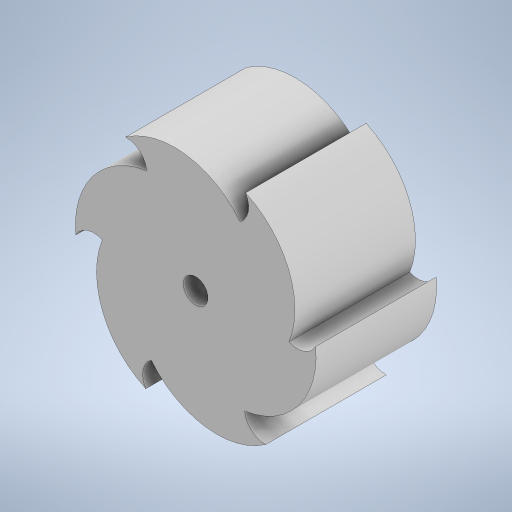
# Autodesk Inventor part: THE_WHEEL
Saved by Autodesk Inventor 2023 (Build 270158000, 158)
## iProperties
Created: 2023-01-26
Part Number: THE_WHEEL
Material: Generic
Document SubType Name: Modeling
Designer: Steven
Density: 1 g/cm^3
Appearance: Default
Author: Steven
Autodesk Inventor part; units mm, degrees
ref_plane "YZ Plane" through (0, 0, 0) normal (1, 0, 0) x (0, 1, 0)
ref_plane "XZ Plane" through (0, 0, 0) normal (0, 1, 0) x (-1, 0, 0)
ref_plane "XY Plane" through (0, 0, 0) normal (0, 0, 1) x (1, 0, 0)
sketch "Sketch1" plane through (0, 0, 0) normal (0, 0, 1) x (1, 0, 0)
  circle A0 centre (0, 0) radius 25.4 construction
  circle A1 centre (0, 0) radius 19.05
  arc A2 (19.0262, -0.952) -> (10.5106, 23.1233) centre (3.175, 6.985) ccw
  arc A3 (8.7227, 16.9357) -> (10.5106, 23.1233) centre (6.8532, 20.828) ccw
  arc A4 (-10.3054, 16.0219) -> (-14.7701, 20.6641) centre (-14.611, 16.349) ccw
  arc A5 (10.3375, 16.0012) -> (-14.7701, 20.6641) centre (-4.4617, 6.2421) ccw
  arc A6 (-19.0281, -0.9138) -> (-25.2807, -2.4592) centre (-21.4642, -4.479) ccw
  arc A7 (-8.6887, 16.9532) -> (-25.2807, -2.4592) centre (-7.6367, -0.7429) ccw
  arc A8 (-8.7227, -16.9357) -> (-10.5106, -23.1233) centre (-6.8532, -20.828) ccw
  arc A9 (-19.0262, 0.952) -> (-10.5106, -23.1233) centre (-3.175, -6.985) ccw
  arc A10 (10.3054, -16.0219) -> (14.7701, -20.6641) centre (14.611, -16.349) ccw
  arc A11 (-10.3375, -16.0012) -> (14.7701, -20.6641) centre (4.4617, -6.2421) ccw
  arc A12 (19.0281, 0.9138) -> (25.2807, 2.4592) centre (21.4642, 4.479) ccw
  arc A13 (8.6887, -16.9532) -> (25.2807, 2.4592) centre (7.6367, 0.7429) ccw
  circle A14 centre (0, 0) radius 2.6035
  point P0 (9.3754, 17.3232)
  point P1 (-10.3146, 16.781)
  point P2 (-19.6901, -0.5423)
  point P3 (-9.3754, -17.3232)
  point P4 (10.3146, -16.781)
  point P5 (19.6901, 0.5423)
  dimension "d0" = 50.8
  dimension "d1" = 38.1
  dimension "d3" = 4.318
  dimension "d4" = 6.985
  dimension "d5" = 3.175
  dimension "d6" = 20.828
  dimension "d9" = 360
  dimension "d11" = 5.207
  constraints: 26 point on circle, 14 centre point, 3 coincident, 47 other
  measures "d1" diameter of A1
  measures "d3" radius of A3
  measures "d4" vertical distance of point (0, 0) A2.centre
  measures "d5" horizontal distance of point (0, 0) A2.centre
  measures "d6" vertical distance of point (0, 0) A3.centre
  measures "d11" diameter of A14
extrude "Extrusion1" add sketch "Sketch1" along normal blind 25.4 contours A1 | A1 A12 A2 | A1 A5 A3 A2 A12 | A2 A12 A13 A10 A1 | A1 A3 A5 | A10 A13 A1 | A1 A7 A4 A5 A3 | A13 A10 A11 A8 A1 | A1 A4 A7 | A8 A11 A1 | A1 A9 A6 A7 A4 | A11 A8 A9 A6 A1 | A1 A6 A9 | A14
extrude "Extrusion2" cut sketch "Sketch1" along normal through all contours A14
body "Solid1"
